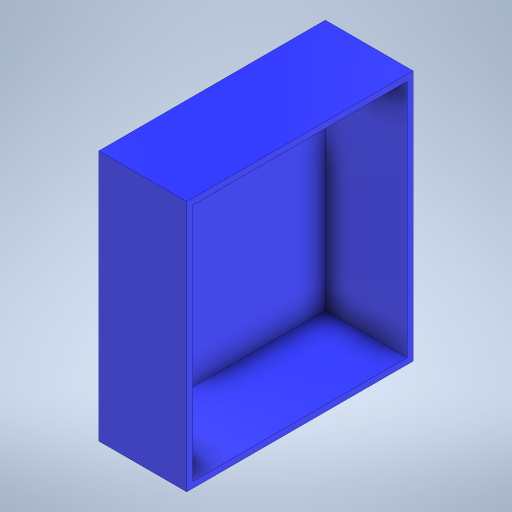
# Autodesk Inventor part: rolling part cabinet
Saved by Autodesk Inventor 2023 (Build 270158000, 158)
## iProperties
Created: 2022-11-15
Part Number: rolling part cabinet
Material: Generic
Document SubType Name: Modeling
Designer: 4026 User
Density: 1 g/cm^3
Appearance: Blue - Wall Paint - Glossy
Author: 4026 User
Autodesk Inventor part; units mm, degrees
ref_plane "YZ Plane" through (0, 0, 0) normal (1, 0, 0) x (0, 1, 0)
ref_plane "XZ Plane" through (0, 0, 0) normal (0, 1, 0) x (-1, 0, 0)
ref_plane "XY Plane" through (0, 0, 0) normal (0, 0, 1) x (1, 0, 0)
sketch "rolling cart" plane through (0, 0, 0) normal (0, 1, 0) x (-1, 0, 0)
  line L0 (368.3, 949.325) -> (0, 949.325)
  line L1 (0, 949.325) -> (0, 0)
  line L2 (0, 0) -> (368.3, 0)
  line L3 (368.3, 0) -> (368.3, 949.325)
  dimension "d0" = 949.325
  dimension "d1" = 368.3
  constraints: 8 end point, 2 parallel, 1 coincident, 1 horizontal, 1 perpendicular
  measures "d0" distance of L2.end L0.start
  measures "d1" distance of L1.end L2.end
extrude "part cabinet" add sketch "rolling cart" along normal blind 1054.1
shell "Shell1" thickness 25.4 removed faces 1 at (0, 351.3667, 632.8833)
body "Solid1"
